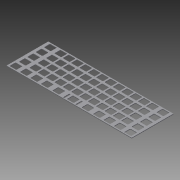
# Autodesk Inventor part: case
Saved by Autodesk Inventor 2015 (Build 190159000, 159)
## iProperties
Created: 2015-07-10
Part Number: case
Material: Generic
Document SubType Name: Modeling
Designer: Ben
Density: 1 g/cm^3
Appearance: Default
Author: Ben
Autodesk Inventor part; units mm, degrees
(part 1 of 2)
ref_plane "YZ Plane" through (0, 0, 0) normal (1, 0, 0) x (0, 1, 0)
ref_plane "XZ Plane" through (0, 0, 0) normal (0, 1, 0) x (-1, 0, 0)
ref_plane "XY Plane" through (0, 0, 0) normal (0, 0, 1) x (1, 0, 0)
sketch "1u" plane through (0, 0, 0) normal (0, 1, 0) x (-1, 0, 0)
  line L0 (7, 7) -> (-7, 7)
  line L1 (-7, 7) -> (-7, 6.4)
  line L2 (-7, 6.4) -> (-7.8, 6.4)
  line L3 (-7.8, 6.4) -> (-7.8, -6.4)
  line L4 (-7.8, -6.4) -> (-7, -6.4)
  line L5 (-7, -6.4) -> (-7, -7)
  line L6 (-7, -7) -> (7, -7)
  line L7 (7, -7) -> (7, -6.4)
  line L8 (7, -6.4) -> (7.8, -6.4)
  line L9 (7.8, -6.4) -> (7.8, 6.4)
  line L10 (7.8, 6.4) -> (7, 6.4)
  line L11 (7, 6.4) -> (7, 7)
  line L12 (9.525, -9.525) -> (9.525, 9.525) construction
  line L13 (9.525, 9.525) -> (-9.525, 9.525) construction
  line L14 (-9.525, 9.525) -> (-9.525, -9.525) construction
  line L15 (-9.525, -9.525) -> (9.525, -9.525) construction
  line L16 (9.525, 0) -> (7.8, 0) construction
  line L17 (-7.8, 0) -> (-9.525, 0) construction
  line L18 (0, 7) -> (0, 9.525) construction
  line L19 (0, -7) -> (0, -9.525) construction
  dimension "d0" = 12.8
  dimension "d1" = 14
  dimension "d2" = 14
  dimension "d3" = 15.6
  dimension "d4" = 19.05
  dimension "d5" = 19.05
  constraints: 40 end point, 14 perpendicular, 8 midpoint, 7 point on line, 6 collinear, 1 horizontal, 1 parallel, 1 vertical
  measures "d0" distance of L8.end L9.end
  measures "d1" distance between parallel lines of L0 L6
  measures "d2" distance of L5.end L6.end
  measures "d3" distance between parallel lines of L3 L9
  measures "d4" distance of L14.end L12.start
  measures "d5" distance of L12.start L12.end
sketch "1.25u" plane through (0, 0, 0) normal (0, 1, 0) x (-1, 0, 0)
  line L0 (7, 7) -> (-7, 7)
  line L1 (-7, 7) -> (-7, 6.4)
  line L2 (-7, 6.4) -> (-7.8, 6.4)
  line L3 (-7.8, 6.4) -> (-7.8, -6.4)
  line L4 (-7.8, -6.4) -> (-7, -6.4)
  line L5 (-7, -6.4) -> (-7, -7)
  line L6 (-7, -7) -> (7, -7)
  line L7 (7, -7) -> (7, -6.4)
  line L8 (7, -6.4) -> (7.8, -6.4)
  line L9 (7.8, -6.4) -> (7.8, 6.4)
  line L10 (7.8, 6.4) -> (7, 6.4)
  line L11 (7, 6.4) -> (7, 7)
  line L12 (11.9063, -9.525) -> (11.9063, 9.525) construction
  line L13 (11.9063, 9.525) -> (-11.9062, 9.525) construction
  line L14 (-11.9062, 9.525) -> (-11.9062, -9.525) construction
  line L15 (-11.9062, -9.525) -> (11.9063, -9.525) construction
  line L16 (11.9062, 0) -> (7.8, 0) construction
  line L17 (-7.8, 0) -> (-11.9062, 0) construction
  line L18 (0, 7) -> (0, 9.525) construction
  line L19 (0, -7) -> (0, -9.525) construction
  dimension "d45" = 12.8
  dimension "d46" = 14
  dimension "d47" = 14
  dimension "d48" = 15.6
  dimension "d49" = 23.8125
  dimension "d50" = 19.05
  constraints: 40 end point, 14 perpendicular, 8 midpoint, 7 point on line, 6 collinear, 1 horizontal, 1 parallel, 1 vertical
  measures "d45" distance of L8.end L9.end
  measures "d46" distance between parallel lines of L0 L6
  measures "d47" distance of L5.end L6.end
  measures "d48" distance between parallel lines of L3 L9
  measures "d49" distance of L14.end L12.start
  measures "d50" distance of L12.start L12.end
sketch "1.5u" plane through (0, 0, 0) normal (0, 1, 0) x (-1, 0, 0)
  line L0 (7, 7) -> (-7, 7)
  line L1 (-7, 7) -> (-7, 6.4)
  line L2 (-7, 6.4) -> (-7.8, 6.4)
  line L3 (-7.8, 6.4) -> (-7.8, -6.4)
  line L4 (-7.8, -6.4) -> (-7, -6.4)
  line L5 (-7, -6.4) -> (-7, -7)
  line L6 (-7, -7) -> (7, -7)
  line L7 (7, -7) -> (7, -6.4)
  line L8 (7, -6.4) -> (7.8, -6.4)
  line L9 (7.8, -6.4) -> (7.8, 6.4)
  line L10 (7.8, 6.4) -> (7, 6.4)
  line L11 (7, 6.4) -> (7, 7)
  line L12 (14.2875, -9.525) -> (14.2875, 9.525) construction
  line L13 (14.2875, 9.525) -> (-14.2875, 9.525) construction
  line L14 (-14.2875, 9.525) -> (-14.2875, -9.525) construction
  line L15 (-14.2875, -9.525) -> (14.2875, -9.525) construction
  line L16 (14.2875, 0) -> (7.8, 0) construction
  line L17 (-7.8, 0) -> (-14.2875, 0) construction
  line L18 (0, 7) -> (0, 9.525) construction
  line L19 (0, -7) -> (0, -9.525) construction
  dimension "d39" = 12.8
  dimension "d40" = 14
  dimension "d41" = 14
  dimension "d42" = 15.6
  dimension "d43" = 28.575
  dimension "d44" = 19.05
  constraints: 40 end point, 14 perpendicular, 8 midpoint, 7 point on line, 6 collinear, 1 horizontal, 1 parallel, 1 vertical
  measures "d39" distance of L8.end L9.end
  measures "d40" distance between parallel lines of L0 L6
  measures "d41" distance of L5.end L6.end
  measures "d42" distance between parallel lines of L3 L9
  measures "d43" distance of L14.end L12.start
  measures "d44" distance of L12.start L12.end
sketch "2u" plane through (0, 0, 0) normal (0, 1, 0) x (-1, 0, 0)
  line L0 (7, -7) -> (7, -6.4)
  line L1 (7, -6.4) -> (7.8, -6.4)
  line L2 (19.05, 0) -> (7.8, 0) construction
  line L3 (19.05, -9.525) -> (19.05, 9.525) construction
  line L4 (7.8, -6.4) -> (7.8, 6.4)
  line L5 (0, -7) -> (0, -9.525) construction
  line L6 (-7, -6.4) -> (-7, -7)
  line L7 (-7.8, 0) -> (-19.05, 0) construction
  line L8 (-7.8, -6.4) -> (-7, -6.4)
  line L9 (0, 7) -> (0, 9.525) construction
  line L10 (7, 7) -> (-7, 7)
  line L11 (-7, -7) -> (7, -7)
  line L12 (-19.05, -9.525) -> (19.05, -9.525) construction
  line L13 (19.05, 9.525) -> (-19.05, 9.525) construction
  line L14 (-19.05, 9.525) -> (-19.05, -9.525) construction
  line L15 (-7, 7) -> (-7, 6.4)
  line L16 (-7, 6.4) -> (-7.8, 6.4)
  line L17 (-7.8, 6.4) -> (-7.8, -6.4)
  line L18 (7, 6.4) -> (7, 7)
  line L19 (7.8, 6.4) -> (7, 6.4)
  line L20 (15.6, -6.24) -> (15.6, 7.76)
  line L21 (15.6, 7.76) -> (12.4, 7.76)
  line L22 (12.4, 7.76) -> (12.4, -6.24)
  line L23 (12.4, -6.24) -> (15.6, -6.24)
  line L24 (14, -6.24) -> (14, 7.76) construction
  line L25 (15.6, 0.76) -> (12.4, 0.76) construction
  line L26 (-12.4, 7.76) -> (-12.4, -6.24)
  line L27 (-12.4, -6.24) -> (-15.6, -6.24)
  line L28 (-15.6, -6.24) -> (-15.6, 7.76)
  line L29 (-15.6, 7.76) -> (-12.4, 7.76)
  line L30 (-14, -6.24) -> (-14, 7.76) construction
  line L31 (-15.6, 0.76) -> (-12.4, 0.76) construction
  dimension "d28" = 12.8
  dimension "d29" = 14
  dimension "d30" = 14
  dimension "d31" = 15.6
  dimension "d32" = 38.1
  dimension "d33" = 19.05
  dimension "d34" = 3.2
  dimension "d35" = 14
  dimension "d36" = 14
  dimension "d37" = 0.76
  constraints: 64 end point, 17 perpendicular, 12 midpoint, 8 symmetric about line, 7 point on line, 6 collinear, 2 vertical, 1 horizontal, 1 parallel
  measures "d28" distance of L4.start L4.end
  measures "d29" distance between parallel lines of L10 L11
  measures "d30" distance of L11.start L0.start
  measures "d31" distance between parallel lines of L17 L4
  measures "d32" distance of L12.start L3.start
  measures "d33" distance of L3.start L3.end
  measures "d34" distance of L22.end L20.start
  measures "d35" distance of L20.start L21.start
  measures "d36" distance between parallel lines of L5 L24
  measures "d37" distance between parallel lines of L25 L2
sketch "Sketch10" plane through (0, 0, 0) normal (0, 1, 0) x (-1, 0, 0)
  line L0 (-4.9062, -2.525) -> (-18.9062, -2.525)
  line L1 (-18.9062, -2.525) -> (-18.9062, -3.125)
  line L2 (-18.9062, -3.125) -> (-19.7062, -3.125)
  line L3 (-19.7062, -3.125) -> (-19.7062, -15.925)
  line L4 (-19.7062, -15.925) -> (-18.9062, -15.925)
  line L5 (-18.9062, -15.925) -> (-18.9062, -16.525)
  line L6 (-18.9062, -16.525) -> (-4.9062, -16.525)
  line L7 (-4.9062, -16.525) -> (-4.9062, -15.925)
  line L8 (-4.9062, -15.925) -> (-4.1062, -15.925)
  line L9 (-4.1062, -15.925) -> (-4.1062, -3.125)
  line L10 (-4.1062, -3.125) -> (-4.9062, -3.125)
  line L11 (-4.9062, -3.125) -> (-4.9062, -2.525)
  line L12 (0, -19.05) -> (0, 0) construction
  line L13 (0, 0) -> (-23.8125, 0) construction
  line L14 (-23.8125, 0) -> (-23.8125, -19.05) construction
  line L15 (-23.8125, -19.05) -> (0, -19.05) construction
  line L16 (0, -9.525) -> (-4.1062, -9.525) construction
  line L17 (-19.7062, -9.525) -> (-23.8125, -9.525) construction
  line L18 (-11.9062, -2.525) -> (-11.9062, 0) construction
  line L19 (-11.9062, -16.525) -> (-11.9062, -19.05) construction
  line L20 (-28.7187, -2.525) -> (-42.7187, -2.525)
  line L21 (-42.7187, -2.525) -> (-42.7187, -3.125)
  line L22 (-42.7187, -3.125) -> (-43.5187, -3.125)
  line L23 (-43.5187, -3.125) -> (-43.5187, -15.925)
  line L24 (-43.5187, -15.925) -> (-42.7187, -15.925)
  line L25 (-42.7187, -15.925) -> (-42.7187, -16.525)
  line L26 (-42.7187, -16.525) -> (-28.7187, -16.525)
  line L27 (-28.7187, -16.525) -> (-28.7187, -15.925)
  line L28 (-28.7187, -15.925) -> (-27.9187, -15.925)
  line L29 (-27.9187, -15.925) -> (-27.9187, -3.125)
  line L30 (-27.9187, -3.125) -> (-28.7187, -3.125)
  line L31 (-28.7187, -3.125) -> (-28.7187, -2.525)
  line L32 (-23.8125, -19.05) -> (-23.8125, 0) construction
  line L33 (-23.8125, 0) -> (-47.625, 0) construction
  line L34 (-47.625, 0) -> (-47.625, -19.05) construction
  line L35 (-47.625, -19.05) -> (-23.8125, -19.05) construction
  line L36 (-23.8125, -9.525) -> (-27.9187, -9.525) construction
  line L37 (-43.5187, -9.525) -> (-47.625, -9.525) construction
  line L38 (-35.7187, -2.525) -> (-35.7187, 0) construction
  line L39 (-35.7187, -16.525) -> (-35.7187, -19.05) construction
  line L40 (-52.5312, -2.525) -> (-66.5312, -2.525)
  line L41 (-66.5312, -2.525) -> (-66.5312, -3.125)
  line L42 (-66.5312, -3.125) -> (-67.3312, -3.125)
  line L43 (-67.3312, -3.125) -> (-67.3312, -15.925)
  line L44 (-67.3312, -15.925) -> (-66.5312, -15.925)
  line L45 (-66.5312, -15.925) -> (-66.5312, -16.525)
  line L46 (-66.5312, -16.525) -> (-52.5312, -16.525)
  line L47 (-52.5312, -16.525) -> (-52.5312, -15.925)
  line L48 (-52.5312, -15.925) -> (-51.7312, -15.925)
  line L49 (-51.7312, -15.925) -> (-51.7312, -3.125)
  line L50 (-51.7312, -3.125) -> (-52.5312, -3.125)
  line L51 (-52.5312, -3.125) -> (-52.5312, -2.525)
  line L52 (-47.625, -19.05) -> (-47.625, 0) construction
  line L53 (-47.625, 0) -> (-71.4375, 0) construction
  line L54 (-71.4375, 0) -> (-71.4375, -19.05) construction
  line L55 (-71.4375, -19.05) -> (-47.625, -19.05) construction
  line L56 (-47.625, -9.525) -> (-51.7312, -9.525) construction
  line L57 (-67.3312, -9.525) -> (-71.4375, -9.525) construction
  line L58 (-59.5312, -2.525) -> (-59.5312, 0) construction
  line L59 (-59.5312, -16.525) -> (-59.5312, -19.05) construction
  line L60 (-76.3437, -2.525) -> (-90.3437, -2.525)
  line L61 (-90.3437, -2.525) -> (-90.3437, -3.125)
  line L62 (-90.3437, -3.125) -> (-91.1437, -3.125)
  line L63 (-91.1437, -3.125) -> (-91.1437, -15.925)
  line L64 (-91.1437, -15.925) -> (-90.3437, -15.925)
  line L65 (-90.3437, -15.925) -> (-90.3437, -16.525)
  line L66 (-90.3437, -16.525) -> (-76.3437, -16.525)
  line L67 (-76.3437, -16.525) -> (-76.3437, -15.925)
  line L68 (-76.3437, -15.925) -> (-75.5437, -15.925)
  line L69 (-75.5437, -15.925) -> (-75.5437, -3.125)
  line L70 (-75.5437, -3.125) -> (-76.3437, -3.125)
  line L71 (-76.3437, -3.125) -> (-76.3437, -2.525)
  line L72 (-71.4375, -19.05) -> (-71.4375, 0) construction
  line L73 (-71.4375, 0) -> (-95.25, 0) construction
  line L74 (-95.25, 0) -> (-95.25, -19.05) construction
  line L75 (-95.25, -19.05) -> (-71.4375, -19.05) construction
  line L76 (-71.4375, -9.525) -> (-75.5437, -9.525) construction
  line L77 (-91.1437, -9.525) -> (-95.25, -9.525) construction
  line L78 (-83.3437, -2.525) -> (-83.3437, 0) construction
  line L79 (-83.3437, -16.525) -> (-83.3437, -19.05) construction
  line L80 (-7.2875, -21.575) -> (-21.2875, -21.575)
  line L81 (-21.2875, -21.575) -> (-21.2875, -22.175)
  line L82 (-21.2875, -22.175) -> (-22.0875, -22.175)
  line L83 (-22.0875, -22.175) -> (-22.0875, -34.975)
  line L84 (-22.0875, -34.975) -> (-21.2875, -34.975)
  line L85 (-21.2875, -34.975) -> (-21.2875, -35.575)
  line L86 (-21.2875, -35.575) -> (-7.2875, -35.575)
  line L87 (-7.2875, -35.575) -> (-7.2875, -34.975)
  line L88 (-7.2875, -34.975) -> (-6.4875, -34.975)
  line L89 (-6.4875, -34.975) -> (-6.4875, -22.175)
  line L90 (-6.4875, -22.175) -> (-7.2875, -22.175)
  line L91 (-7.2875, -22.175) -> (-7.2875, -21.575)
  line L92 (0, -38.1) -> (0, -19.05) construction
  line L93 (0, -19.05) -> (-28.575, -19.05) construction
  line L94 (-28.575, -19.05) -> (-28.575, -38.1) construction
  line L95 (-28.575, -38.1) -> (0, -38.1) construction
  line L96 (0, -28.575) -> (-6.4875, -28.575) construction
  line L97 (-22.0875, -28.575) -> (-28.575, -28.575) construction
  line L98 (-14.2875, -21.575) -> (-14.2875, -19.05) construction
  line L99 (-14.2875, -35.575) -> (-14.2875, -38.1) construction
  line L100 (-7.2875, -40.625) -> (-21.2875, -40.625)
  line L101 (-21.2875, -40.625) -> (-21.2875, -41.225)
  line L102 (-21.2875, -41.225) -> (-22.0875, -41.225)
  line L103 (-22.0875, -41.225) -> (-22.0875, -54.025)
  line L104 (-22.0875, -54.025) -> (-21.2875, -54.025)
  line L105 (-21.2875, -54.025) -> (-21.2875, -54.625)
  line L106 (-21.2875, -54.625) -> (-7.2875, -54.625)
  line L107 (-7.2875, -54.625) -> (-7.2875, -54.025)
  line L108 (-7.2875, -54.025) -> (-6.4875, -54.025)
  line L109 (-6.4875, -54.025) -> (-6.4875, -41.225)
  line L110 (-6.4875, -41.225) -> (-7.2875, -41.225)
  line L111 (-7.2875, -41.225) -> (-7.2875, -40.625)
  line L112 (0, -57.15) -> (0, -38.1) construction
  line L113 (0, -38.1) -> (-28.575, -38.1) construction
  line L114 (-28.575, -38.1) -> (-28.575, -57.15) construction
  line L115 (-28.575, -57.15) -> (0, -57.15) construction
  line L116 (0, -47.625) -> (-6.4875, -47.625) construction
  line L117 (-22.0875, -47.625) -> (-28.575, -47.625) construction
  line L118 (-14.2875, -40.625) -> (-14.2875, -38.1) construction
  line L119 (-14.2875, -54.625) -> (-14.2875, -57.15) construction
  line L120 (-7.2875, -59.675) -> (-21.2875, -59.675)
  line L121 (-21.2875, -59.675) -> (-21.2875, -60.275)
  line L122 (-21.2875, -60.275) -> (-22.0875, -60.275)
  line L123 (-22.0875, -60.275) -> (-22.0875, -73.075)
  line L124 (-22.0875, -73.075) -> (-21.2875, -73.075)
  line L125 (-21.2875, -73.075) -> (-21.2875, -73.675)
  line L126 (-21.2875, -73.675) -> (-7.2875, -73.675)
  line L127 (-7.2875, -73.675) -> (-7.2875, -73.075)
  line L128 (-7.2875, -73.075) -> (-6.4875, -73.075)
  line L129 (-6.4875, -73.075) -> (-6.4875, -60.275)
  line L130 (-6.4875, -60.275) -> (-7.2875, -60.275)
  line L131 (-7.2875, -60.275) -> (-7.2875, -59.675)
  line L132 (0, -76.2) -> (0, -57.15) construction
  line L133 (0, -57.15) -> (-28.575, -57.15) construction
  line L134 (-28.575, -57.15) -> (-28.575, -76.2) construction
  line L135 (-28.575, -76.2) -> (0, -76.2) construction
  line L136 (0, -66.675) -> (-6.4875, -66.675) construction
  line L137 (-22.0875, -66.675) -> (-28.575, -66.675) construction
  line L138 (-14.2875, -59.675) -> (-14.2875, -57.15) construction
  line L139 (-14.2875, -73.675) -> (-14.2875, -76.2) construction
  line L140 (-7.2875, -78.725) -> (-21.2875, -78.725)
  line L141 (-21.2875, -78.725) -> (-21.2875, -79.325)
  line L142 (-21.2875, -79.325) -> (-22.0875, -79.325)
  line L143 (-22.0875, -79.325) -> (-22.0875, -92.125)
  line L144 (-22.0875, -92.125) -> (-21.2875, -92.125)
  line L145 (-21.2875, -92.125) -> (-21.2875, -92.725)
  line L146 (-21.2875, -92.725) -> (-7.2875, -92.725)
  line L147 (-7.2875, -92.725) -> (-7.2875, -92.125)
  line L148 (-7.2875, -92.125) -> (-6.4875, -92.125)
  line L149 (-6.4875, -92.125) -> (-6.4875, -79.325)
  line L150 (-6.4875, -79.325) -> (-7.2875, -79.325)
  line L151 (-7.2875, -79.325) -> (-7.2875, -78.725)
  line L152 (0, -95.25) -> (0, -76.2) construction
  line L153 (0, -76.2) -> (-28.575, -76.2) construction
  line L154 (-28.575, -76.2) -> (-28.575, -95.25) construction
  line L155 (-28.575, -95.25) -> (0, -95.25) construction
  line L156 (0, -85.725) -> (-6.4875, -85.725) construction
  line L157 (-22.0875, -85.725) -> (-28.575, -85.725) construction
  line L158 (-14.2875, -78.725) -> (-14.2875, -76.2) construction
  line L159 (-14.2875, -92.725) -> (-14.2875, -95.25) construction
  line L160 (-31.1, -21.575) -> (-45.1, -21.575)
  line L161 (-45.1, -21.575) -> (-45.1, -22.175)
  line L162 (-45.1, -22.175) -> (-45.9, -22.175)
  line L163 (-45.9, -22.175) -> (-45.9, -34.975)
  line L164 (-45.9, -34.975) -> (-45.1, -34.975)
  line L165 (-45.1, -34.975) -> (-45.1, -35.575)
  line L166 (-45.1, -35.575) -> (-31.1, -35.575)
  line L167 (-31.1, -35.575) -> (-31.1, -34.975)
  line L168 (-31.1, -34.975) -> (-30.3, -34.975)
  line L169 (-30.3, -34.975) -> (-30.3, -22.175)
  line L170 (-30.3, -22.175) -> (-31.1, -22.175)
  line L171 (-31.1, -22.175) -> (-31.1, -21.575)
  line L172 (-28.575, -38.1) -> (-28.575, -19.05) construction
  line L173 (-28.575, -19.05) -> (-47.625, -19.05) construction
  line L174 (-47.625, -19.05) -> (-47.625, -38.1) construction
  line L175 (-47.625, -38.1) -> (-28.575, -38.1) construction
  line L176 (-28.575, -28.575) -> (-30.3, -28.575) construction
  line L177 (-45.9, -28.575) -> (-47.625, -28.575) construction
  line L178 (-38.1, -21.575) -> (-38.1, -19.05) construction
  line L179 (-38.1, -35.575) -> (-38.1, -38.1) construction
  line L180 (-31.1, -40.625) -> (-45.1, -40.625)
  line L181 (-45.1, -40.625) -> (-45.1, -41.225)
  line L182 (-45.1, -41.225) -> (-45.9, -41.225)
  line L183 (-45.9, -41.225) -> (-45.9, -54.025)
  line L184 (-45.9, -54.025) -> (-45.1, -54.025)
  line L185 (-45.1, -54.025) -> (-45.1, -54.625)
  line L186 (-45.1, -54.625) -> (-31.1, -54.625)
  line L187 (-31.1, -54.625) -> (-31.1, -54.025)
  line L188 (-31.1, -54.025) -> (-30.3, -54.025)
  line L189 (-30.3, -54.025) -> (-30.3, -41.225)
  line L190 (-30.3, -41.225) -> (-31.1, -41.225)
  line L191 (-31.1, -41.225) -> (-31.1, -40.625)
  line L192 (-28.575, -57.15) -> (-28.575, -38.1) construction
  line L193 (-28.575, -38.1) -> (-47.625, -38.1) construction
  line L194 (-47.625, -38.1) -> (-47.625, -57.15) construction
  line L195 (-47.625, -57.15) -> (-28.575, -57.15) construction
  line L196 (-28.575, -47.625) -> (-30.3, -47.625) construction
  line L197 (-45.9, -47.625) -> (-47.625, -47.625) construction
  line L198 (-38.1, -40.625) -> (-38.1, -38.1) construction
  line L199 (-38.1, -54.625) -> (-38.1, -57.15) construction
  line L200 (-31.1, -59.675) -> (-45.1, -59.675)
  line L201 (-45.1, -59.675) -> (-45.1, -60.275)
  line L202 (-45.1, -60.275) -> (-45.9, -60.275)
  line L203 (-45.9, -60.275) -> (-45.9, -73.075)
  line L204 (-45.9, -73.075) -> (-45.1, -73.075)
  line L205 (-45.1, -73.075) -> (-45.1, -73.675)
  line L206 (-45.1, -73.675) -> (-31.1, -73.675)
  line L207 (-31.1, -73.675) -> (-31.1, -73.075)
  line L208 (-31.1, -73.075) -> (-30.3, -73.075)
  line L209 (-30.3, -73.075) -> (-30.3, -60.275)
  line L210 (-30.3, -60.275) -> (-31.1, -60.275)
  line L211 (-31.1, -60.275) -> (-31.1, -59.675)
  line L212 (-28.575, -76.2) -> (-28.575, -57.15) construction
  line L213 (-28.575, -57.15) -> (-47.625, -57.15) construction
  line L214 (-47.625, -57.15) -> (-47.625, -76.2) construction
  line L215 (-47.625, -76.2) -> (-28.575, -76.2) construction
  line L216 (-28.575, -66.675) -> (-30.3, -66.675) construction
  line L217 (-45.9, -66.675) -> (-47.625, -66.675) construction
  line L218 (-38.1, -59.675) -> (-38.1, -57.15) construction
  line L219 (-38.1, -73.675) -> (-38.1, -76.2) construction
  line L220 (-31.1, -78.725) -> (-45.1, -78.725)
  line L221 (-45.1, -78.725) -> (-45.1, -79.325)
  line L222 (-45.1, -79.325) -> (-45.9, -79.325)
  line L223 (-45.9, -79.325) -> (-45.9, -92.125)
  line L224 (-45.9, -92.125) -> (-45.1, -92.125)
  line L225 (-45.1, -92.125) -> (-45.1, -92.725)
  line L226 (-45.1, -92.725) -> (-31.1, -92.725)
  line L227 (-31.1, -92.725) -> (-31.1, -92.125)
  line L228 (-31.1, -92.125) -> (-30.3, -92.125)
  line L229 (-30.3, -92.125) -> (-30.3, -79.325)
  line L230 (-30.3, -79.325) -> (-31.1, -79.325)
  line L231 (-31.1, -79.325) -> (-31.1, -78.725)
  line L232 (-28.575, -95.25) -> (-28.575, -76.2) construction
  line L233 (-28.575, -76.2) -> (-47.625, -76.2) construction
  line L234 (-47.625, -76.2) -> (-47.625, -95.25) construction
  line L235 (-47.625, -95.25) -> (-28.575, -95.25) construction
  line L236 (-28.575, -85.725) -> (-30.3, -85.725) construction
  line L237 (-45.9, -85.725) -> (-47.625, -85.725) construction
  line L238 (-38.1, -78.725) -> (-38.1, -76.2) construction
  line L239 (-38.1, -92.725) -> (-38.1, -95.25) construction
  line L240 (-50.15, -21.575) -> (-64.15, -21.575)
  line L241 (-64.15, -21.575) -> (-64.15, -22.175)
  line L242 (-64.15, -22.175) -> (-64.95, -22.175)
  line L243 (-64.95, -22.175) -> (-64.95, -34.975)
  line L244 (-64.95, -34.975) -> (-64.15, -34.975)
  line L245 (-64.15, -34.975) -> (-64.15, -35.575)
  line L246 (-64.15, -35.575) -> (-50.15, -35.575)
  line L247 (-50.15, -35.575) -> (-50.15, -34.975)
  line L248 (-50.15, -34.975) -> (-49.35, -34.975)
  line L249 (-49.35, -34.975) -> (-49.35, -22.175)
  line L250 (-49.35, -22.175) -> (-50.15, -22.175)
  line L251 (-50.15, -22.175) -> (-50.15, -21.575)
  line L252 (-47.625, -38.1) -> (-47.625, -19.05) construction
  line L253 (-47.625, -19.05) -> (-66.675, -19.05) construction
  line L254 (-66.675, -19.05) -> (-66.675, -38.1) construction
  line L255 (-66.675, -38.1) -> (-47.625, -38.1) construction
  line L256 (-47.625, -28.575) -> (-49.35, -28.575) construction
  line L257 (-64.95, -28.575) -> (-66.675, -28.575) construction
  line L258 (-57.15, -21.575) -> (-57.15, -19.05) construction
  line L259 (-57.15, -35.575) -> (-57.15, -38.1) construction
  line L260 (-50.15, -40.625) -> (-64.15, -40.625)
  line L261 (-64.15, -40.625) -> (-64.15, -41.225)
  line L262 (-64.15, -41.225) -> (-64.95, -41.225)
  line L263 (-64.95, -41.225) -> (-64.95, -54.025)
  line L264 (-64.95, -54.025) -> (-64.15, -54.025)
  line L265 (-64.15, -54.025) -> (-64.15, -54.625)
  line L266 (-64.15, -54.625) -> (-50.15, -54.625)
  line L267 (-50.15, -54.625) -> (-50.15, -54.025)
  line L268 (-50.15, -54.025) -> (-49.35, -54.025)
  line L269 (-49.35, -54.025) -> (-49.35, -41.225)
  line L270 (-49.35, -41.225) -> (-50.15, -41.225)
  line L271 (-50.15, -41.225) -> (-50.15, -40.625)
  line L272 (-47.625, -57.15) -> (-47.625, -38.1) construction
  line L273 (-47.625, -38.1) -> (-66.675, -38.1) construction
  line L274 (-66.675, -38.1) -> (-66.675, -57.15) construction
  line L275 (-66.675, -57.15) -> (-47.625, -57.15) construction
  line L276 (-47.625, -47.625) -> (-49.35, -47.625) construction
  line L277 (-64.95, -47.625) -> (-66.675, -47.625) construction
  line L278 (-57.15, -40.625) -> (-57.15, -38.1) construction
  line L279 (-57.15, -54.625) -> (-57.15, -57.15) construction
  line L280 (-50.15, -59.675) -> (-64.15, -59.675)
  line L281 (-64.15, -59.675) -> (-64.15, -60.275)
  line L282 (-64.15, -60.275) -> (-64.95, -60.275)
  line L283 (-64.95, -60.275) -> (-64.95, -73.075)
  line L284 (-64.95, -73.075) -> (-64.15, -73.075)
  line L285 (-64.15, -73.075) -> (-64.15, -73.675)
  line L286 (-64.15, -73.675) -> (-50.15, -73.675)
  line L287 (-50.15, -73.675) -> (-50.15, -73.075)
  line L288 (-50.15, -73.075) -> (-49.35, -73.075)
  line L289 (-49.35, -73.075) -> (-49.35, -60.275)
  line L290 (-49.35, -60.275) -> (-50.15, -60.275)
  line L291 (-50.15, -60.275) -> (-50.15, -59.675)
  line L292 (-47.625, -76.2) -> (-47.625, -57.15) construction
  line L293 (-47.625, -57.15) -> (-66.675, -57.15) construction
  line L294 (-66.675, -57.15) -> (-66.675, -76.2) construction
  line L295 (-66.675, -76.2) -> (-47.625, -76.2) construction
  line L296 (-47.625, -66.675) -> (-49.35, -66.675) construction
  line L297 (-64.95, -66.675) -> (-66.675, -66.675) construction
  line L298 (-57.15, -59.675) -> (-57.15, -57.15) construction
  line L299 (-57.15, -73.675) -> (-57.15, -76.2) construction
  line L300 (-50.15, -78.725) -> (-64.15, -78.725)
  line L301 (-64.15, -78.725) -> (-64.15, -79.325)
  line L302 (-64.15, -79.325) -> (-64.95, -79.325)
  line L303 (-64.95, -79.325) -> (-64.95, -92.125)
  line L304 (-64.95, -92.125) -> (-64.15, -92.125)
  line L305 (-64.15, -92.125) -> (-64.15, -92.725)
  line L306 (-64.15, -92.725) -> (-50.15, -92.725)
  line L307 (-50.15, -92.725) -> (-50.15, -92.125)
  line L308 (-50.15, -92.125) -> (-49.35, -92.125)
  line L309 (-49.35, -92.125) -> (-49.35, -79.325)
  line L310 (-49.35, -79.325) -> (-50.15, -79.325)
  line L311 (-50.15, -79.325) -> (-50.15, -78.725)
  line L312 (-47.625, -95.25) -> (-47.625, -76.2) construction
  line L313 (-47.625, -76.2) -> (-66.675, -76.2) construction
  line L314 (-66.675, -76.2) -> (-66.675, -95.25) construction
  line L315 (-66.675, -95.25) -> (-47.625, -95.25) construction
  line L316 (-47.625, -85.725) -> (-49.35, -85.725) construction
  line L317 (-64.95, -85.725) -> (-66.675, -85.725) construction
  line L318 (-57.15, -78.725) -> (-57.15, -76.2) construction
  line L319 (-57.15, -92.725) -> (-57.15, -95.25) construction
  line L320 (-69.2, -21.575) -> (-83.2, -21.575)
  line L321 (-83.2, -21.575) -> (-83.2, -22.175)
  line L322 (-83.2, -22.175) -> (-84, -22.175)
  line L323 (-84, -22.175) -> (-84, -34.975)
  line L324 (-84, -34.975) -> (-83.2, -34.975)
  line L325 (-83.2, -34.975) -> (-83.2, -35.575)
  line L326 (-83.2, -35.575) -> (-69.2, -35.575)
  line L327 (-69.2, -35.575) -> (-69.2, -34.975)
  line L328 (-69.2, -34.975) -> (-68.4, -34.975)
  line L329 (-68.4, -34.975) -> (-68.4, -22.175)
  line L330 (-68.4, -22.175) -> (-69.2, -22.175)
  line L331 (-69.2, -22.175) -> (-69.2, -21.575)
  line L332 (-66.675, -38.1) -> (-66.675, -19.05) construction
  line L333 (-66.675, -19.05) -> (-85.725, -19.05) construction
  line L334 (-85.725, -19.05) -> (-85.725, -38.1) construction
  line L335 (-85.725, -38.1) -> (-66.675, -38.1) construction
  line L336 (-66.675, -28.575) -> (-68.4, -28.575) construction
  line L337 (-84, -28.575) -> (-85.725, -28.575) construction
  line L338 (-76.2, -21.575) -> (-76.2, -19.05) construction
  line L339 (-76.2, -35.575) -> (-76.2, -38.1) construction
  line L340 (-69.2, -40.625) -> (-83.2, -40.625)
  line L341 (-83.2, -40.625) -> (-83.2, -41.225)
  line L342 (-83.2, -41.225) -> (-84, -41.225)
  line L343 (-84, -41.225) -> (-84, -54.025)
  line L344 (-84, -54.025) -> (-83.2, -54.025)
  line L345 (-83.2, -54.025) -> (-83.2, -54.625)
  line L346 (-83.2, -54.625) -> (-69.2, -54.625)
  line L347 (-69.2, -54.625) -> (-69.2, -54.025)
  line L348 (-69.2, -54.025) -> (-68.4, -54.025)
  line L349 (-68.4, -54.025) -> (-68.4, -41.225)
  line L350 (-68.4, -41.225) -> (-69.2, -41.225)
  line L351 (-69.2, -41.225) -> (-69.2, -40.625)
  line L352 (-66.675, -57.15) -> (-66.675, -38.1) construction
  line L353 (-66.675, -38.1) -> (-85.725, -38.1) construction
  line L354 (-85.725, -38.1) -> (-85.725, -57.15) construction
  line L355 (-85.725, -57.15) -> (-66.675, -57.15) construction
  line L356 (-66.675, -47.625) -> (-68.4, -47.625) construction
  line L357 (-84, -47.625) -> (-85.725, -47.625) construction
  line L358 (-76.2, -40.625) -> (-76.2, -38.1) construction
  line L359 (-76.2, -54.625) -> (-76.2, -57.15) construction
  line L360 (-69.2, -59.675) -> (-83.2, -59.675)
  line L361 (-83.2, -59.675) -> (-83.2, -60.275)
  line L362 (-83.2, -60.275) -> (-84, -60.275)
  line L363 (-84, -60.275) -> (-84, -73.075)
  line L364 (-84, -73.075) -> (-83.2, -73.075)
  line L365 (-83.2, -73.075) -> (-83.2, -73.675)
  line L366 (-83.2, -73.675) -> (-69.2, -73.675)
  line L367 (-69.2, -73.675) -> (-69.2, -73.075)
  line L368 (-69.2, -73.075) -> (-68.4, -73.075)
  line L369 (-68.4, -73.075) -> (-68.4, -60.275)
  line L370 (-68.4, -60.275) -> (-69.2, -60.275)
  line L371 (-69.2, -60.275) -> (-69.2, -59.675)
  line L372 (-66.675, -76.2) -> (-66.675, -57.15) construction
  line L373 (-66.675, -57.15) -> (-85.725, -57.15) construction
  line L374 (-85.725, -57.15) -> (-85.725, -76.2) construction
  line L375 (-85.725, -76.2) -> (-66.675, -76.2) construction
  line L376 (-66.675, -66.675) -> (-68.4, -66.675) construction
  line L377 (-84, -66.675) -> (-85.725, -66.675) construction
  line L378 (-76.2, -59.675) -> (-76.2, -57.15) construction
  line L379 (-76.2, -73.675) -> (-76.2, -76.2) construction
  line L380 (-69.2, -78.725) -> (-83.2, -78.725)
  line L381 (-83.2, -78.725) -> (-83.2, -79.325)
  line L382 (-83.2, -79.325) -> (-84, -79.325)
  line L383 (-84, -79.325) -> (-84, -92.125)
  line L384 (-84, -92.125) -> (-83.2, -92.125)
  line L385 (-83.2, -92.125) -> (-83.2, -92.725)
  line L386 (-83.2, -92.725) -> (-69.2, -92.725)
  line L387 (-69.2, -92.725) -> (-69.2, -92.125)
  line L388 (-69.2, -92.125) -> (-68.4, -92.125)
  line L389 (-68.4, -92.125) -> (-68.4, -79.325)
  line L390 (-68.4, -79.325) -> (-69.2, -79.325)
  line L391 (-69.2, -79.325) -> (-69.2, -78.725)
  line L392 (-66.675, -95.25) -> (-66.675, -76.2) construction
  line L393 (-66.675, -76.2) -> (-85.725, -76.2) construction
  line L394 (-85.725, -76.2) -> (-85.725, -95.25) construction
  line L395 (-85.725, -95.25) -> (-66.675, -95.25) construction
  line L396 (-66.675, -85.725) -> (-68.4, -85.725) construction
  line L397 (-84, -85.725) -> (-85.725, -85.725) construction
  line L398 (-76.2, -78.725) -> (-76.2, -76.2) construction
  line L399 (-76.2, -92.725) -> (-76.2, -95.25) construction
  line L400 (-88.25, -21.575) -> (-102.25, -21.575)
  line L401 (-102.25, -21.575) -> (-102.25, -22.175)
  line L402 (-102.25, -22.175) -> (-103.05, -22.175)
  line L403 (-103.05, -22.175) -> (-103.05, -34.975)
  line L404 (-103.05, -34.975) -> (-102.25, -34.975)
  line L405 (-102.25, -34.975) -> (-102.25, -35.575)
  line L406 (-102.25, -35.575) -> (-88.25, -35.575)
  line L407 (-88.25, -35.575) -> (-88.25, -34.975)
  line L408 (-88.25, -34.975) -> (-87.45, -34.975)
  line L409 (-87.45, -34.975) -> (-87.45, -22.175)
  line L410 (-87.45, -22.175) -> (-88.25, -22.175)
  line L411 (-88.25, -22.175) -> (-88.25, -21.575)
  line L412 (-85.725, -38.1) -> (-85.725, -19.05) construction
  line L413 (-85.725, -19.05) -> (-104.775, -19.05) construction
  line L414 (-104.775, -19.05) -> (-104.775, -38.1) construction
  line L415 (-104.775, -38.1) -> (-85.725, -38.1) construction
  line L416 (-85.725, -28.575) -> (-87.45, -28.575) construction
  line L417 (-103.05, -28.575) -> (-104.775, -28.575) construction
  line L418 (-95.25, -21.575) -> (-95.25, -19.05) construction
  line L419 (-95.25, -35.575) -> (-95.25, -38.1) construction
  line L420 (-88.25, -40.625) -> (-102.25, -40.625)
  line L421 (-102.25, -40.625) -> (-102.25, -41.225)
  line L422 (-102.25, -41.225) -> (-103.05, -41.225)
  line L423 (-103.05, -41.225) -> (-103.05, -54.025)
  line L424 (-103.05, -54.025) -> (-102.25, -54.025)
  line L425 (-102.25, -54.025) -> (-102.25, -54.625)
  line L426 (-102.25, -54.625) -> (-88.25, -54.625)
  line L427 (-88.25, -54.625) -> (-88.25, -54.025)
  line L428 (-88.25, -54.025) -> (-87.45, -54.025)
  line L429 (-87.45, -54.025) -> (-87.45, -41.225)
  line L430 (-87.45, -41.225) -> (-88.25, -41.225)
  line L431 (-88.25, -41.225) -> (-88.25, -40.625)
  line L432 (-85.725, -57.15) -> (-85.725, -38.1) construction
  line L433 (-85.725, -38.1) -> (-104.775, -38.1) construction
  line L434 (-104.775, -38.1) -> (-104.775, -57.15) construction
  line L435 (-104.775, -57.15) -> (-85.725, -57.15) construction
  line L436 (-85.725, -47.625) -> (-87.45, -47.625) construction
  line L437 (-103.05, -47.625) -> (-104.775, -47.625) construction
  line L438 (-95.25, -40.625) -> (-95.25, -38.1) construction
  line L439 (-95.25, -54.625) -> (-95.25, -57.15) construction
  line L440 (-88.25, -59.675) -> (-102.25, -59.675)
  line L441 (-102.25, -59.675) -> (-102.25, -60.275)
  line L442 (-102.25, -60.275) -> (-103.05, -60.275)
  line L443 (-103.05, -60.275) -> (-103.05, -73.075)
  line L444 (-103.05, -73.075) -> (-102.25, -73.075)
  line L445 (-102.25, -73.075) -> (-102.25, -73.675)
  line L446 (-102.25, -73.675) -> (-88.25, -73.675)
  line L447 (-88.25, -73.675) -> (-88.25, -73.075)
  line L448 (-88.25, -73.075) -> (-87.45, -73.075)
  line L449 (-87.45, -73.075) -> (-87.45, -60.275)
  line L450 (-87.45, -60.275) -> (-88.25, -60.275)
  line L451 (-88.25, -60.275) -> (-88.25, -59.675)
  line L452 (-85.725, -76.2) -> (-85.725, -57.15) construction
  line L453 (-85.725, -57.15) -> (-104.775, -57.15) construction
  line L454 (-104.775, -57.15) -> (-104.775, -76.2) construction
  line L455 (-104.775, -76.2) -> (-85.725, -76.2) construction
  line L456 (-85.725, -66.675) -> (-87.45, -66.675) construction
  line L457 (-103.05, -66.675) -> (-104.775, -66.675) construction
  line L458 (-95.25, -59.675) -> (-95.25, -57.15) construction
  line L459 (-95.25, -73.675) -> (-95.25, -76.2) construction
  line L460 (-88.25, -78.725) -> (-102.25, -78.725)
  line L461 (-102.25, -78.725) -> (-102.25, -79.325)
  line L462 (-102.25, -79.325) -> (-103.05, -79.325)
  line L463 (-103.05, -79.325) -> (-103.05, -92.125)
  line L464 (-103.05, -92.125) -> (-102.25, -92.125)
  line L465 (-102.25, -92.125) -> (-102.25, -92.725)
  line L466 (-102.25, -92.725) -> (-88.25, -92.725)
  line L467 (-88.25, -92.725) -> (-88.25, -92.125)
  line L468 (-88.25, -92.125) -> (-87.45, -92.125)
  line L469 (-87.45, -92.125) -> (-87.45, -79.325)
  line L470 (-87.45, -79.325) -> (-88.25, -79.325)
  line L471 (-88.25, -79.325) -> (-88.25, -78.725)
  line L472 (-85.725, -95.25) -> (-85.725, -76.2) construction
  line L473 (-85.725, -76.2) -> (-104.775, -76.2) construction
  line L474 (-104.775, -76.2) -> (-104.775, -95.25) construction
  line L475 (-104.775, -95.25) -> (-85.725, -95.25) construction
  line L476 (-85.725, -85.725) -> (-87.45, -85.725) construction
  line L477 (-103.05, -85.725) -> (-104.775, -85.725) construction
  line L478 (-95.25, -78.725) -> (-95.25, -76.2) construction
  line L479 (-95.25, -92.725) -> (-95.25, -95.25) construction
  line L480 (-107.3, -21.575) -> (-121.3, -21.575)
  line L481 (-121.3, -21.575) -> (-121.3, -22.175)
  line L482 (-121.3, -22.175) -> (-122.1, -22.175)
  line L483 (-122.1, -22.175) -> (-122.1, -34.975)
  line L484 (-122.1, -34.975) -> (-121.3, -34.975)
  line L485 (-121.3, -34.975) -> (-121.3, -35.575)
  line L486 (-121.3, -35.575) -> (-107.3, -35.575)
  line L487 (-107.3, -35.575) -> (-107.3, -34.975)
  line L488 (-107.3, -34.975) -> (-106.5, -34.975)
  line L489 (-106.5, -34.975) -> (-106.5, -22.175)
  line L490 (-106.5, -22.175) -> (-107.3, -22.175)
  line L491 (-107.3, -22.175) -> (-107.3, -21.575)
  line L492 (-104.775, -38.1) -> (-104.775, -19.05) construction
  line L493 (-104.775, -19.05) -> (-123.825, -19.05) construction
  line L494 (-123.825, -19.05) -> (-123.825, -38.1) construction
  line L495 (-123.825, -38.1) -> (-104.775, -38.1) construction
  line L496 (-104.775, -28.575) -> (-106.5, -28.575) construction
  line L497 (-122.1, -28.575) -> (-123.825, -28.575) construction
  line L498 (-114.3, -21.575) -> (-114.3, -19.05) construction
  line L499 (-114.3, -35.575) -> (-114.3, -38.1) construction
  line L500 (-107.3, -40.625) -> (-121.3, -40.625)
  line L501 (-121.3, -40.625) -> (-121.3, -41.225)
  line L502 (-121.3, -41.225) -> (-122.1, -41.225)
  line L503 (-122.1, -41.225) -> (-122.1, -54.025)
  line L504 (-122.1, -54.025) -> (-121.3, -54.025)
  line L505 (-121.3, -54.025) -> (-121.3, -54.625)
  line L506 (-121.3, -54.625) -> (-107.3, -54.625)
  line L507 (-107.3, -54.625) -> (-107.3, -54.025)
  line L508 (-107.3, -54.025) -> (-106.5, -54.025)
  line L509 (-106.5, -54.025) -> (-106.5, -41.225)
  line L510 (-106.5, -41.225) -> (-107.3, -41.225)
  line L511 (-107.3, -41.225) -> (-107.3, -40.625)
  line L512 (-104.775, -57.15) -> (-104.775, -38.1) construction
  line L513 (-104.775, -38.1) -> (-123.825, -38.1) construction
  line L514 (-123.825, -38.1) -> (-123.825, -57.15) construction
  line L515 (-123.825, -57.15) -> (-104.775, -57.15) construction
  line L516 (-104.775, -47.625) -> (-106.5, -47.625) construction
  line L517 (-122.1, -47.625) -> (-123.825, -47.625) construction
  line L518 (-114.3, -40.625) -> (-114.3, -38.1) construction
  line L519 (-114.3, -54.625) -> (-114.3, -57.15) construction
  line L520 (-107.3, -59.675) -> (-121.3, -59.675)
  line L521 (-121.3, -59.675) -> (-121.3, -60.275)
  line L522 (-121.3, -60.275) -> (-122.1, -60.275)
  line L523 (-122.1, -60.275) -> (-122.1, -73.075)
  line L524 (-122.1, -73.075) -> (-121.3, -73.075)
  line L525 (-121.3, -73.075) -> (-121.3, -73.675)
  line L526 (-121.3, -73.675) -> (-107.3, -73.675)
  line L527 (-107.3, -73.675) -> (-107.3, -73.075)
  line L528 (-107.3, -73.075) -> (-106.5, -73.075)
  line L529 (-106.5, -73.075) -> (-106.5, -60.275)
  line L530 (-106.5, -60.275) -> (-107.3, -60.275)
  line L531 (-107.3, -60.275) -> (-107.3, -59.675)
  line L532 (-104.775, -76.2) -> (-104.775, -57.15) construction
  line L533 (-104.775, -57.15) -> (-123.825, -57.15) construction
  line L534 (-123.825, -57.15) -> (-123.825, -76.2) construction
  line L535 (-123.825, -76.2) -> (-104.775, -76.2) construction
  line L536 (-104.775, -66.675) -> (-106.5, -66.675) construction
  line L537 (-122.1, -66.675) -> (-123.825, -66.675) construction
  line L538 (-114.3, -59.675) -> (-114.3, -57.15) construction
  line L539 (-114.3, -73.675) -> (-114.3, -76.2) construction
  line L540 (-107.3, -78.725) -> (-121.3, -78.725)
  line L541 (-121.3, -78.725) -> (-121.3, -79.325)
  line L542 (-121.3, -79.325) -> (-122.1, -79.325)
  line L543 (-122.1, -79.325) -> (-122.1, -92.125)
  line L544 (-122.1, -92.125) -> (-121.3, -92.125)
  line L545 (-121.3, -92.125) -> (-121.3, -92.725)
  line L546 (-121.3, -92.725) -> (-107.3, -92.725)
  line L547 (-107.3, -92.725) -> (-107.3, -92.125)
  line L548 (-107.3, -92.125) -> (-106.5, -92.125)
  line L549 (-106.5, -92.125) -> (-106.5, -79.325)
  line L550 (-106.5, -79.325) -> (-107.3, -79.325)
  line L551 (-107.3, -79.325) -> (-107.3, -78.725)
  line L552 (-104.775, -95.25) -> (-104.775, -76.2) construction
  line L553 (-104.775, -76.2) -> (-123.825, -76.2) construction
  line L554 (-123.825, -76.2) -> (-123.825, -95.25) construction
  line L555 (-123.825, -95.25) -> (-104.775, -95.25) construction
  line L556 (-104.775, -85.725) -> (-106.5, -85.725) construction
  line L557 (-122.1, -85.725) -> (-123.825, -85.725) construction
  line L558 (-114.3, -78.725) -> (-114.3, -76.2) construction
  line L559 (-114.3, -92.725) -> (-114.3, -95.25) construction
  line L560 (-126.35, -21.575) -> (-140.35, -21.575)
  line L561 (-140.35, -21.575) -> (-140.35, -22.175)
  line L562 (-140.35, -22.175) -> (-141.15, -22.175)
  line L563 (-141.15, -22.175) -> (-141.15, -34.975)
  line L564 (-141.15, -34.975) -> (-140.35, -34.975)
  line L565 (-140.35, -34.975) -> (-140.35, -35.575)
  line L566 (-140.35, -35.575) -> (-126.35, -35.575)
  line L567 (-126.35, -35.575) -> (-126.35, -34.975)
  line L568 (-126.35, -34.975) -> (-125.55, -34.975)
  line L569 (-125.55, -34.975) -> (-125.55, -22.175)
  line L570 (-125.55, -22.175) -> (-126.35, -22.175)
  line L571 (-126.35, -22.175) -> (-126.35, -21.575)
  line L572 (-123.825, -38.1) -> (-123.825, -19.05) construction
  line L573 (-123.825, -19.05) -> (-142.875, -19.05) construction
  line L574 (-142.875, -19.05) -> (-142.875, -38.1) construction
  line L575 (-142.875, -38.1) -> (-123.825, -38.1) construction
  line L576 (-123.825, -28.575) -> (-125.55, -28.575) construction
  line L577 (-141.15, -28.575) -> (-142.875, -28.575) construction
  line L578 (-133.35, -21.575) -> (-133.35, -19.05) construction
  line L579 (-133.35, -35.575) -> (-133.35, -38.1) construction
  line L580 (-126.35, -40.625) -> (-140.35, -40.625)
  line L581 (-140.35, -40.625) -> (-140.35, -41.225)
  line L582 (-140.35, -41.225) -> (-141.15, -41.225)
  line L583 (-141.15, -41.225) -> (-141.15, -54.025)
  line L584 (-141.15, -54.025) -> (-140.35, -54.025)
  line L585 (-140.35, -54.025) -> (-140.35, -54.625)
  line L586 (-140.35, -54.625) -> (-126.35, -54.625)
  line L587 (-126.35, -54.625) -> (-126.35, -54.025)
  line L588 (-126.35, -54.025) -> (-125.55, -54.025)
  line L589 (-125.55, -54.025) -> (-125.55, -41.225)
  line L590 (-125.55, -41.225) -> (-126.35, -41.225)
  line L591 (-126.35, -41.225) -> (-126.35, -40.625)
  line L592 (-123.825, -57.15) -> (-123.825, -38.1) construction
  line L593 (-123.825, -38.1) -> (-142.875, -38.1) construction
  line L594 (-142.875, -38.1) -> (-142.875, -57.15) construction
  line L595 (-142.875, -57.15) -> (-123.825, -57.15) construction
  line L596 (-123.825, -47.625) -> (-125.55, -47.625) construction
  line L597 (-141.15, -47.625) -> (-142.875, -47.625) construction
  line L598 (-133.35, -40.625) -> (-133.35, -38.1) construction
  line L599 (-133.35, -54.625) -> (-133.35, -57.15) construction
  line L600 (-126.35, -59.675) -> (-140.35, -59.675)
  line L601 (-140.35, -59.675) -> (-140.35, -60.275)
  line L602 (-140.35, -60.275) -> (-141.15, -60.275)
  line L603 (-141.15, -60.275) -> (-141.15, -73.075)
  line L604 (-141.15, -73.075) -> (-140.35, -73.075)
  line L605 (-140.35, -73.075) -> (-140.35, -73.675)
  line L606 (-140.35, -73.675) -> (-126.35, -73.675)
  line L607 (-126.35, -73.675) -> (-126.35, -73.075)
  line L608 (-126.35, -73.075) -> (-125.55, -73.075)
  line L609 (-125.55, -73.075) -> (-125.55, -60.275)
  line L610 (-125.55, -60.275) -> (-126.35, -60.275)
  line L611 (-126.35, -60.275) -> (-126.35, -59.675)
  line L612 (-123.825, -76.2) -> (-123.825, -57.15) construction
  line L613 (-123.825, -57.15) -> (-142.875, -57.15) construction
  line L614 (-142.875, -57.15) -> (-142.875, -76.2) construction
  line L615 (-142.875, -76.2) -> (-123.825, -76.2) construction
  line L616 (-123.825, -66.675) -> (-125.55, -66.675) construction
  line L617 (-141.15, -66.675) -> (-142.875, -66.675) construction
  line L618 (-133.35, -59.675) -> (-133.35, -57.15) construction
  line L619 (-133.35, -73.675) -> (-133.35, -76.2) construction
  line L620 (-126.35, -78.725) -> (-140.35, -78.725)
  line L621 (-140.35, -78.725) -> (-140.35, -79.325)
  line L622 (-140.35, -79.325) -> (-141.15, -79.325)
  line L623 (-141.15, -79.325) -> (-141.15, -92.125)
  line L624 (-141.15, -92.125) -> (-140.35, -92.125)
  line L625 (-140.35, -92.125) -> (-140.35, -92.725)
  line L626 (-140.35, -92.725) -> (-126.35, -92.725)
  line L627 (-126.35, -92.725) -> (-126.35, -92.125)
  line L628 (-126.35, -92.125) -> (-125.55, -92.125)
  line L629 (-125.55, -92.125) -> (-125.55, -79.325)
  line L630 (-125.55, -79.325) -> (-126.35, -79.325)
  line L631 (-126.35, -79.325) -> (-126.35, -78.725)
  line L632 (-123.825, -95.25) -> (-123.825, -76.2) construction
  line L633 (-123.825, -76.2) -> (-142.875, -76.2) construction
  line L634 (-142.875, -76.2) -> (-142.875, -95.25) construction
  line L635 (-142.875, -95.25) -> (-123.825, -95.25) construction
  line L636 (-123.825, -85.725) -> (-125.55, -85.725) construction
  line L637 (-141.15, -85.725) -> (-142.875, -85.725) construction
  line L638 (-133.35, -78.725) -> (-133.35, -76.2) construction
  line L639 (-133.35, -92.725) -> (-133.35, -95.25) construction
  line L640 (-145.4, -21.575) -> (-159.4, -21.575)
  line L641 (-159.4, -21.575) -> (-159.4, -22.175)
  line L642 (-159.4, -22.175) -> (-160.2, -22.175)
  line L643 (-160.2, -22.175) -> (-160.2, -34.975)
  line L644 (-160.2, -34.975) -> (-159.4, -34.975)
  line L645 (-159.4, -34.975) -> (-159.4, -35.575)
  line L646 (-159.4, -35.575) -> (-145.4, -35.575)
  line L647 (-145.4, -35.575) -> (-145.4, -34.975)
  line L648 (-145.4, -34.975) -> (-144.6, -34.975)
  line L649 (-144.6, -34.975) -> (-144.6, -22.175)
  line L650 (-144.6, -22.175) -> (-145.4, -22.175)
  line L651 (-145.4, -22.175) -> (-145.4, -21.575)
  line L652 (-142.875, -38.1) -> (-142.875, -19.05) construction
  line L653 (-142.875, -19.05) -> (-161.925, -19.05) construction
  line L654 (-161.925, -19.05) -> (-161.925, -38.1) construction
  line L655 (-161.925, -38.1) -> (-142.875, -38.1) construction
  line L656 (-142.875, -28.575) -> (-144.6, -28.575) construction
  line L657 (-160.2, -28.575) -> (-161.925, -28.575) construction
  line L658 (-152.4, -21.575) -> (-152.4, -19.05) construction
  line L659 (-152.4, -35.575) -> (-152.4, -38.1) construction
  line L660 (-145.4, -40.625) -> (-159.4, -40.625)
  line L661 (-159.4, -40.625) -> (-159.4, -41.225)
  line L662 (-159.4, -41.225) -> (-160.2, -41.225)
  line L663 (-160.2, -41.225) -> (-160.2, -54.025)
  line L664 (-160.2, -54.025) -> (-159.4, -54.025)
  line L665 (-159.4, -54.025) -> (-159.4, -54.625)
  line L666 (-159.4, -54.625) -> (-145.4, -54.625)
  line L667 (-145.4, -54.625) -> (-145.4, -54.025)
  line L668 (-145.4, -54.025) -> (-144.6, -54.025)
  line L669 (-144.6, -54.025) -> (-144.6, -41.225)
  line L670 (-144.6, -41.225) -> (-145.4, -41.225)
  line L671 (-145.4, -41.225) -> (-145.4, -40.625)
  line L672 (-142.875, -57.15) -> (-142.875, -38.1) construction
  line L673 (-142.875, -38.1) -> (-161.925, -38.1) construction
  line L674 (-161.925, -38.1) -> (-161.925, -57.15) construction
  line L675 (-161.925, -57.15) -> (-142.875, -57.15) construction
  line L676 (-142.875, -47.625) -> (-144.6, -47.625) construction
  line L677 (-160.2, -47.625) -> (-161.925, -47.625) construction
  line L678 (-152.4, -40.625) -> (-152.4, -38.1) construction
  line L679 (-152.4, -54.625) -> (-152.4, -57.15) construction
  line L680 (-145.4, -59.675) -> (-159.4, -59.675)
  line L681 (-159.4, -59.675) -> (-159.4, -60.275)
  line L682 (-159.4, -60.275) -> (-160.2, -60.275)
  line L683 (-160.2, -60.275) -> (-160.2, -73.075)
  line L684 (-160.2, -73.075) -> (-159.4, -73.075)
  line L685 (-159.4, -73.075) -> (-159.4, -73.675)
  line L686 (-159.4, -73.675) -> (-145.4, -73.675)
  line L687 (-145.4, -73.675) -> (-145.4, -73.075)
  line L688 (-145.4, -73.075) -> (-144.6, -73.075)
  line L689 (-144.6, -73.075) -> (-144.6, -60.275)
  line L690 (-144.6, -60.275) -> (-145.4, -60.275)
  line L691 (-145.4, -60.275) -> (-145.4, -59.675)
  line L692 (-142.875, -76.2) -> (-142.875, -57.15) construction
  line L693 (-142.875, -57.15) -> (-161.925, -57.15) construction
  line L694 (-161.925, -57.15) -> (-161.925, -76.2) construction
  line L695 (-161.925, -76.2) -> (-142.875, -76.2) construction
  line L696 (-142.875, -66.675) -> (-144.6, -66.675) construction
  line L697 (-160.2, -66.675) -> (-161.925, -66.675) construction
  line L698 (-152.4, -59.675) -> (-152.4, -57.15) construction
  line L699 (-152.4, -73.675) -> (-152.4, -76.2) construction
  line L700 (-145.4, -78.725) -> (-159.4, -78.725)
  line L701 (-159.4, -78.725) -> (-159.4, -79.325)
  line L702 (-159.4, -79.325) -> (-160.2, -79.325)
  line L703 (-160.2, -79.325) -> (-160.2, -92.125)
  line L704 (-160.2, -92.125) -> (-159.4, -92.125)
  line L705 (-159.4, -92.125) -> (-159.4, -92.725)
  line L706 (-159.4, -92.725) -> (-145.4, -92.725)
  line L707 (-145.4, -92.725) -> (-145.4, -92.125)
  line L708 (-145.4, -92.125) -> (-144.6, -92.125)
  line L709 (-144.6, -92.125) -> (-144.6, -79.325)
  line L710 (-144.6, -79.325) -> (-145.4, -79.325)
  line L711 (-145.4, -79.325) -> (-145.4, -78.725)
  line L712 (-142.875, -95.25) -> (-142.875, -76.2) construction
  line L713 (-142.875, -76.2) -> (-161.925, -76.2) construction
  line L714 (-161.925, -76.2) -> (-161.925, -95.25) construction
  line L715 (-161.925, -95.25) -> (-142.875, -95.25) construction
  line L716 (-142.875, -85.725) -> (-144.6, -85.725) construction
  line L717 (-160.2, -85.725) -> (-161.925, -85.725) construction
  line L718 (-152.4, -78.725) -> (-152.4, -76.2) construction
  line L719 (-152.4, -92.725) -> (-152.4, -95.25) construction
  line L720 (-164.45, -21.575) -> (-178.45, -21.575)
  line L721 (-178.45, -21.575) -> (-178.45, -22.175)
  line L722 (-178.45, -22.175) -> (-179.25, -22.175)
  line L723 (-179.25, -22.175) -> (-179.25, -34.975)
  line L724 (-179.25, -34.975) -> (-178.45, -34.975)
  line L725 (-178.45, -34.975) -> (-178.45, -35.575)
  line L726 (-178.45, -35.575) -> (-164.45, -35.575)
  line L727 (-164.45, -35.575) -> (-164.45, -34.975)
  line L728 (-164.45, -34.975) -> (-163.65, -34.975)
  line L729 (-163.65, -34.975) -> (-163.65, -22.175)
  line L730 (-163.65, -22.175) -> (-164.45, -22.175)
  line L731 (-164.45, -22.175) -> (-164.45, -21.575)
  line L732 (-161.925, -38.1) -> (-161.925, -19.05) construction
  line L733 (-161.925, -19.05) -> (-180.975, -19.05) construction
  line L734 (-180.975, -19.05) -> (-180.975, -38.1) construction
  line L735 (-180.975, -38.1) -> (-161.925, -38.1) construction
  line L736 (-161.925, -28.575) -> (-163.65, -28.575) construction
  line L737 (-179.25, -28.575) -> (-180.975, -28.575) construction
  line L738 (-171.45, -21.575) -> (-171.45, -19.05) construction
  line L739 (-171.45, -35.575) -> (-171.45, -38.1) construction
  line L740 (-164.45, -40.625) -> (-178.45, -40.625)
  line L741 (-178.45, -40.625) -> (-178.45, -41.225)
  line L742 (-178.45, -41.225) -> (-179.25, -41.225)
  line L743 (-179.25, -41.225) -> (-179.25, -54.025)
  line L744 (-179.25, -54.025) -> (-178.45, -54.025)
  line L745 (-178.45, -54.025) -> (-178.45, -54.625)
  line L746 (-178.45, -54.625) -> (-164.45, -54.625)
  line L747 (-164.45, -54.625) -> (-164.45, -54.025)
  line L748 (-164.45, -54.025) -> (-163.65, -54.025)
  line L749 (-163.65, -54.025) -> (-163.65, -41.225)
  line L750 (-163.65, -41.225) -> (-164.45, -41.225)
  line L751 (-164.45, -41.225) -> (-164.45, -40.625)
  line L752 (-161.925, -57.15) -> (-161.925, -38.1) construction
  line L753 (-161.925, -38.1) -> (-180.975, -38.1) construction
  line L754 (-180.975, -38.1) -> (-180.975, -57.15) construction
  line L755 (-180.975, -57.15) -> (-161.925, -57.15) construction
  line L756 (-161.925, -47.625) -> (-163.65, -47.625) construction
  line L757 (-179.25, -47.625) -> (-180.975, -47.625) construction
  line L758 (-171.45, -40.625) -> (-171.45, -38.1) construction